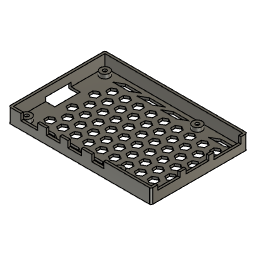
Raspberry pi 4B Case 01 (Autodesk Fusion 360 design; units mm, degrees)
Autodesk Fusion 360 part; units mm, degrees
sketch "スケッチ1" plane through (0, 0, 0) normal (0, 0, 1) x (1, 0, 0)
  line L0 (2.2, 2.2) -> (87.2, 2.2) construction
  line L1 (87.2, 2.2) -> (87.2, 58.2) construction
  line L2 (87.2, 58.2) -> (2.2, 58.2) construction
  line L3 (5.7, 5.7) -> (63.7, 5.7) construction
  line L4 (63.7, 5.7) -> (63.7, 54.7) construction
  line L5 (63.7, 54.7) -> (5.7, 54.7) construction
  line L6 (5.7, 54.7) -> (5.7, 5.7) construction
  circle A0 centre (5.7, 54.7) radius 1.15
  circle A1 centre (63.7, 54.7) radius 1.15
  circle A2 centre (63.7, 5.7) radius 1.15
  circle A3 centre (5.7, 5.7) radius 1.15
  line L7 (2.2, 58.2) -> (2.2, 2.2) construction
  line L8 (0, 0) -> (89.4, 0)
  line L9 (89.4, 0) -> (89.4, 60.4)
  line L10 (89.4, 60.4) -> (0, 60.4)
  line L11 (0, 60.4) -> (0, 0)
  line L12 (1.5, 58.9) -> (87.9, 58.9)
  line L13 (87.9, 58.9) -> (87.9, 1.5)
  line L14 (87.9, 1.5) -> (1.5, 1.5)
  line L15 (1.5, 1.5) -> (1.5, 58.9)
  circle A4 centre (5.7, 54.7) radius 3
  circle A5 centre (63.7, 54.7) radius 3
  circle A6 centre (63.7, 5.7) radius 3
  circle A7 centre (5.7, 5.7) radius 3
  line L16 (8.2, 0.7) -> (17.7, 0.7) construction
  line L17 (17.7, 0.7) -> (17.7, 9.7) construction
  line L18 (17.7, 9.7) -> (8.2, 9.7) construction
  line L19 (8.2, 9.7) -> (8.2, 0.7) construction
  line L20 (7.7, 1.5) -> (7.7, 0)
  line L21 (18.2, 1.5) -> (18.2, 0)
  line L22 (24.2, 0.7) -> (31.7, 0.7) construction
  line L23 (31.7, 0.7) -> (31.7, 9.7) construction
  line L24 (31.7, 9.7) -> (24.2, 9.7) construction
  line L25 (24.2, 9.7) -> (24.2, 0.7) construction
  line L26 (45.2, 0.7) -> (45.2, 9.7) construction
  line L27 (37.7, 0.7) -> (45.2, 0.7) construction
  line L28 (45.2, 9.7) -> (37.7, 9.7) construction
  line L29 (37.7, 9.7) -> (37.7, 0.7) construction
  line L30 (23.7, 1.5) -> (23.7, 0)
  line L31 (37.2, 1.5) -> (37.2, 0)
  line L32 (32.2, 1.5) -> (32.2, 0)
  line L33 (45.7, 1.5) -> (45.7, 0)
  line L34 (52.7, 0.2) -> (59.2, 0.2) construction
  line L35 (59.2, 0.2) -> (59.2, 15.2) construction
  line L36 (59.2, 15.2) -> (52.7, 15.2) construction
  line L37 (52.7, 15.2) -> (52.7, 0.2) construction
  line L38 (90.2, 4.7) -> (72.7, 4.7) construction
  line L39 (90.2, 17.7) -> (90.2, 4.7) construction
  line L40 (72.7, 4.7) -> (72.7, 17.7) construction
  line L41 (72.7, 17.7) -> (90.2, 17.7) construction
  line L42 (90.2, 35.7) -> (72.7, 35.7) construction
  line L43 (90.2, 22.7) -> (90.2, 35.7) construction
  line L44 (72.7, 35.7) -> (72.7, 22.7) construction
  line L45 (72.7, 22.7) -> (90.2, 22.7) construction
  line L46 (52.2, 1.5) -> (52.2, 0)
  line L47 (59.7, 1.5) -> (59.7, 0)
  line L48 (69.2, 39.95) -> (90.2, 39.95) construction
  line L49 (90.2, 55.95) -> (69.2, 55.95) construction
  line L50 (69.2, 55.95) -> (69.2, 39.95) construction
  line L51 (90.2, 39.95) -> (90.2, 55.95) construction
  line L52 (81.45, 17.7) -> (81.45, 4.7) construction
  line L53 (72.7, 11.2) -> (90.2, 11.2) construction
  line L54 (81.45, 35.7) -> (81.45, 22.7) construction
  line L55 (72.7, 29.2) -> (90.2, 29.2) construction
  line L56 (79.7, 55.95) -> (79.7, 39.95) construction
  line L57 (69.2, 47.95) -> (90.2, 47.95) construction
  line L58 (87.9, 4.2) -> (89.4, 4.2)
  line L59 (87.9, 18.2) -> (89.4, 18.2)
  line L60 (87.9, 21.9659) -> (89.4, 21.9659)
  line L61 (87.9, 36.2) -> (89.4, 36.2)
  line L62 (89.4, 39.45) -> (87.9, 39.45)
  line L63 (87.9, 56.45) -> (89.4, 56.45)
  line L64 (4.2, 35.7) -> (15.7, 35.7) construction
  line L65 (15.7, 35.7) -> (15.7, 23.7) construction
  line L66 (15.7, 23.7) -> (4.2, 23.7) construction
  line L67 (4.2, 23.7) -> (4.2, 35.7) construction
  line L68 (0, 37.7) -> (7.2, 37.7)
  line L69 (7.2, 37.7) -> (7.2, 21.7)
  line L70 (7.2, 21.7) -> (0, 21.7)
  circle A8 centre (5.7, 5.7) radius 2
  circle A9 centre (63.7, 5.7) radius 2
  circle A10 centre (63.7, 54.7) radius 2
  circle A11 centre (5.7, 54.7) radius 2
  dimension "d1" = 49
  dimension "d2" = 58
  dimension "d3" = 2.3
  dimension "d5" = 3.5
  dimension "d7" = 56
  dimension "d8" = 85
  dimension "d9" = 3.5
  dimension "d10" = 0.7
  dimension "d11" = 0.7
  dimension "d12" = 0.7
  dimension "d13" = 0.7
  dimension "d14" = 1.5
  dimension "d15" = 1.5
  dimension "d16" = 1.5
  dimension "d17" = 1.5
  dimension "d18" = 6
  dimension "d19" = 6
  dimension "d20" = 15.5
  dimension "d21" = 9
  dimension "d22" = 1.5
  dimension "d23" = 0.5
  dimension "d24" = 0.5
  dimension "d25" = 22
  dimension "d26" = 29.5
  dimension "d27" = 35.5
  dimension "d28" = 43
  dimension "d29" = 1.5
  dimension "d30" = 1.5
  dimension "d31" = 0.5
  dimension "d32" = 0.5
  dimension "d33" = 0.5
  dimension "d34" = 0.5
  dimension "d35" = 50.5
  dimension "d36" = 57
  dimension "d37" = 15
  dimension "d38" = 2
  dimension "d39" = 0.5
  dimension "d40" = 0.5
  dimension "d41" = 6.5
  dimension "d42" = 7.5
  dimension "d43" = 9.5
  dimension "d44" = 7.5
  dimension "d46" = 13
  dimension "d47" = 16
  dimension "d48" = 9
  dimension "d49" = 27
  dimension "d50" = 45.75
  dimension "d51" = 21
  dimension "d52" = 17.5
  dimension "d53" = 3
  dimension "d54" = 3
  dimension "d55" = 3
  dimension "d56" = 0.5
  dimension "d57" = 0.5
  dimension "d58" = 0.5
  dimension "d59" = 0.5
  dimension "d60" = 0.5
  dimension "d61" = 0.7341
  dimension "d62" = 21.5
  dimension "d63" = 11.5
  dimension "d64" = 12
  dimension "d65" = 2
  dimension "d66" = 2
  dimension "d67" = 2
  dimension "d68" = 3
  dimension "d84" = 60.4
  dimension "d85" = 89.4
  dimension "d127" = 4
  constraint horizontal L0
  constraint vertical L1
  constraint horizontal L2
  constraint horizontal L3
  constraint vertical L4
  constraint horizontal L5
  constraint vertical L6
  constraint coincident L5.end L6.start
  constraint coincident L4.end L5.start
  constraint coincident L3.end L4.start
  constraint coincident L3.start L6.end
  constraint equal A0 A3
  constraint equal A0 A1
  constraint equal A1 A2
  constraint vertical L7
  constraint horizontal L8
  constraint vertical L9
  constraint horizontal L10
  constraint vertical L11
  constraint coincident L8.start L11.end
  constraint horizontal L12
  constraint vertical L13
  constraint horizontal L14
  constraint vertical L15
  constraint concentric A0 A4
  constraint concentric A1 A5
  constraint concentric A2 A6
  constraint concentric A3 A7
  constraint equal A4 A7
  constraint equal A4 A5
  constraint equal A5 A6
  constraint horizontal L16
  constraint vertical L17
  constraint horizontal L18
  constraint vertical L19
  constraint coincident L14 L20.start
  constraint coincident L8 L20.end
  constraint perpendicular L8 L20
  constraint coincident L14 L21.start
  constraint coincident L8 L21.end
  constraint perpendicular L8 L21
  constraint horizontal L22
  constraint vertical L23
  constraint horizontal L24
  constraint vertical L25
  constraint horizontal L27
  constraint vertical L26
  constraint horizontal L28
  constraint vertical L29
  constraint equal L17 L23
  constraint equal L23 L26
  constraint coincident L14 L30.start
  constraint coincident L8 L30.end
  constraint perpendicular L8 L30
  constraint coincident L14 L31.start
  constraint coincident L8 L31.end
  constraint perpendicular L8 L31
  constraint coincident L14 L32.start
  constraint coincident L8 L32.end
  constraint perpendicular L14 L32
  constraint coincident L14 L33.start
  constraint coincident L8 L33.end
  constraint perpendicular L8 L33
  constraint horizontal L34
  constraint vertical L35
  constraint horizontal L36
  constraint vertical L37
  constraint horizontal L38
  constraint vertical L40
  constraint horizontal L41
  constraint vertical L39
  constraint horizontal L42
  constraint vertical L44
  constraint horizontal L45
  constraint vertical L43
  constraint coincident L14 L46.start
  constraint coincident L8 L46.end
  constraint perpendicular L8 L46
  constraint coincident L14 L47.start
  constraint coincident L8 L47.end
  constraint perpendicular L8 L47
  constraint horizontal L49
  constraint vertical L50
  constraint horizontal L48
  constraint vertical L51
  constraint midpoint L41 L52.start
  constraint midpoint L38 L52.end
  constraint coincident L40 L53.start
  constraint perpendicular L40 L53
  constraint midpoint L52 L53
  constraint midpoint L42 L54.start
  constraint midpoint L45 L54.end
  constraint coincident L44 L55.start
  constraint coincident L43 L55.end
  constraint perpendicular L43 L55
  constraint midpoint L49 L56.start
  constraint midpoint L48 L56.end
  constraint coincident L50 L57.start
  constraint coincident L51 L57.end
  constraint perpendicular L51 L57
  constraint midpoint L56 L57
  constraint midpoint L54 L55
  constraint equal L40 L44
  constraint equal L41 L45
  constraint coincident L13 L58.start
  constraint coincident L9 L58.end
  constraint perpendicular L9 L58
  constraint coincident L13 L59.start
  constraint coincident L9 L59.end
  constraint perpendicular L9 L59
  constraint coincident L13 L60.start
  constraint coincident L9 L60.end
  constraint perpendicular L9 L60
  constraint coincident L13 L61.start
  constraint coincident L9 L61.end
  constraint perpendicular L9 L61
  constraint coincident L9 L62.start
  constraint coincident L13 L62.end
  constraint perpendicular L9 L62
  constraint coincident L13 L63.start
  constraint coincident L9 L63.end
  constraint perpendicular L9 L63
  constraint horizontal L64
  constraint vertical L65
  constraint horizontal L66
  constraint vertical L67
  constraint coincident L11 L68.start
  constraint perpendicular L15 L68
  constraint perpendicular L66 L69
  constraint coincident L11 L70.end
  constraint perpendicular L11 L70
  constraint concentric A7 A8
  constraint concentric A2 A9
  constraint concentric A5 A10
  constraint concentric A0 A11
  constraint equal A8 A9
  constraint equal A9 A10
  constraint equal A10 A11
  measures "d1" distance of L3.start L5.end
  measures "d2" distance of L4.end L5.end
  measures "d3" diameter of A0
  measures "d5" distance of L2 L5
  measures "d7" distance of L0.end L1.end
  measures "d8" distance of L0.end L0.start
  measures "d9" distance of L6 L7
  measures "d10" distance of L2 L12
  measures "d11" distance of L7 L15
  measures "d12" distance of L0 L14
  measures "d13" distance of L1 L13
  measures "d14" distance of L10 L12
  measures "d15" distance of L11 L15
  measures "d16" distance of L9 L13
  measures "d17" distance of L8 L14
  measures "d18" diameter of A4
  measures "d19" distance of L7 L19
  measures "d20" distance of L7 L17
  measures "d21" distance of L16.end L17.end
  measures "d22" distance of L0 L16
  measures "d23" distance of L19 L20
  measures "d24" distance of L17 L21
  measures "d25" distance of L7 L25
  measures "d26" distance of L7 L23
  measures "d27" distance of L7 L29
  measures "d28" distance of L7 L26
  measures "d29" distance of L0 L22
  measures "d30" distance of L0 L27
  measures "d31" distance of L25 L30.start
  measures "d32" distance of L23 L32.start
  measures "d33" distance of L29 L31.start
  measures "d34" distance of L26 L33.start
  measures "d35" distance of L7 L37
  measures "d36" distance of L7 L35
  measures "d37" distance of L34.end L35.end
  measures "d38" distance of L0 L34
  measures "d39" distance of L37 L46
  measures "d40" distance of L35 L47
  measures "d41" distance of L35 L37
  measures "d42" distance of L26 L29
  measures "d43" distance of L17 L19
  measures "d44" distance of L23 L25
  measures "d46" distance of L42 L45
  measures "d47" distance of L48 L49
  measures "d48" distance of L0 L53
  measures "d49" distance of L0 L55
  measures "d50" distance of L0 L57
  measures "d51" distance of L49.start L49.end
  measures "d52" distance of L42.end L42.start
  measures "d53" distance of L1 L39
  measures "d54" distance of L1 L43
  measures "d55" distance of L1 L51
  measures "d56" distance of L41 L59
  measures "d57" distance of L38 L58
  measures "d58" distance of L49 L63
  measures "d59" distance of L48 L62
  measures "d60" distance of L42 L61
  measures "d61" distance of L45 L60
  measures "d62" distance of L0 L66
  measures "d63" distance of L65.end L66.end
  measures "d64" distance of L64 L66
  measures "d65" distance of L7 L67
  measures "d66" distance of L64 L68
  measures "d67" distance of L66 L70
  measures "d68" distance of L67 L69
  measures "d84" distance of L8 L10
  measures "d85" distance of L9 L11
  measures "d127" diameter of A11
extrude "押し出し1" add sketch "スケッチ1" along normal blind 1.5 contours L8 L11 L14 L15 L20 L70 | L8 L14 L20 L21 | L8 L14 L21 L30 | L12 L13 L14 L15 L68 L69 L70 | L9 L10 L11 L12 L13 L15 L63 L68 | L8 L14 L30 L32 | L8 L14 L31 L32 | L8 L14 L31 L33 | L9 L13 L62 L63 | L8 L14 L33 L46 | L9 L13 L61 L62 | L8 L14 L46 L47 | L9 L13 L60 L61 | L8 L9 L13 L14 L47 L58 | L9 L13 L59 L60 | L9 L13 L58 L59 | A4 | A5 | A6 | A7 | A8 | A9 | A10 | A11
extrude "押し出し2" add sketch "スケッチ1" along normal blind 4 contours A4 | A5 | A6 | A7 | A8 | A9 | A10 | A11
extrude "押し出し3" add sketch "スケッチ1" along normal blind 5 contours L8 L11 L14 L15 L20 L70 | L8 L14 L20 L21 | L8 L14 L21 L30 | L9 L10 L11 L12 L13 L15 L63 L68 | L8 L14 L30 L32 | L8 L14 L31 L32 | L8 L14 L31 L33 | L9 L13 L62 L63 | L8 L14 L33 L46 | L9 L13 L61 L62 | L8 L14 L46 L47 | L9 L13 L60 L61 | L8 L9 L13 L14 L47 L58 | L9 L13 L59 L60 | L9 L13 L58 L59
extrude "押し出し4" add sketch "スケッチ1" along normal blind 6 contours L8 L11 L14 L15 L20 L70 | L8 L14 L21 L30 | L9 L10 L11 L12 L13 L15 L63 L68 | L8 L14 L31 L32 | L8 L14 L33 L46 | L9 L13 L61 L62 | L9 L13 L60 L61 | L8 L9 L13 L14 L47 L58 | L9 L13 L59 L60 | L9 L13 L58 L59
extrude "押し出し5" add sketch "スケッチ1" along normal blind 5 from surface at 4 contours L11 L15 L68 L70
extrude "押し出し6" add sketch "スケッチ1" along normal blind 9 contours L8 L11 L14 L15 L20 L70 | L8 L14 L21 L30 | L9 L10 L11 L12 L13 L15 L63 L68 | L8 L14 L31 L32 | L8 L14 L33 L46 | L9 L13 L61 L62 | L8 L9 L13 L14 L47 L58 | L9 L13 L59 L60
fillet "フィレット1" radius 1 4 edges at (89.4, 60.4, 4.5) (89.4, 0, 4.5) (0, 60.4, 4.5) (0, 0, 4.5)
sketch "スケッチ2" plane through (0, 0, 0) normal (0, 0, 1) x (1, 0, 0)
  line L0 (0, 0) -> (89.4, 0) construction
  line L1 (89.4, 0) -> (89.4, 60.4) construction
  line L2 (89.4, 60.4) -> (0, 60.4) construction
  line L3 (0, 60.4) -> (0, 0) construction
  line L4 (10.5, 11.5566) -> (13, 10.1132)
  line L5 (10.5, 14.4434) -> (10.5, 11.5566)
  line L6 (15.5, 11.5566) -> (15.5, 14.4434)
  line L7 (13, 10.1132) -> (15.5, 11.5566)
  line L8 (15.5, 14.4434) -> (13, 15.8868)
  line L9 (13, 15.8868) -> (10.5, 14.4434)
  line L10 (17, 22.8868) -> (14.5, 21.4434)
  line L11 (14.5, 18.5566) -> (17, 17.1132)
  line L12 (14.5, 18.5566) -> (17, 17.1132)
  line L13 (19.5, 18.5566) -> (19.5, 21.4434)
  line L14 (14.5, 21.4434) -> (14.5, 18.5566)
  line L15 (19.5, 21.4434) -> (17, 22.8868)
  line L16 (17, 22.8868) -> (14.5, 21.4434)
  line L17 (14.5, 21.4434) -> (14.5, 18.5566)
  line L18 (17, 17.1132) -> (19.5, 18.5566)
  line L19 (19.5, 18.5566) -> (19.5, 21.4434)
  line L20 (19.5, 21.4434) -> (17, 22.8868)
  line L21 (17, 17.1132) -> (19.5, 18.5566)
  line L22 (13, 13) -> (17, 13) construction
  line L23 (17, 13) -> (17, 20) construction
  line L24 (17, 20) -> (13, 20) construction
  line L25 (13, 20) -> (13, 13) construction
  line L26 (21.125, 10.1132) -> (23.625, 11.5566)
  line L27 (18.625, 11.5566) -> (21.125, 10.1132)
  line L28 (18.625, 14.4434) -> (18.625, 11.5566)
  line L29 (21.125, 15.8868) -> (18.625, 14.4434)
  line L30 (23.625, 14.4434) -> (21.125, 15.8868)
  line L31 (23.625, 11.5566) -> (23.625, 14.4434)
  line L32 (22.625, 18.5566) -> (25.125, 17.1132)
  line L33 (22.625, 21.4434) -> (22.625, 18.5566)
  line L34 (25.125, 22.8868) -> (22.625, 21.4434)
  line L35 (27.625, 21.4434) -> (25.125, 22.8868)
  line L36 (27.625, 18.5566) -> (27.625, 21.4434)
  line L37 (25.125, 17.1132) -> (27.625, 18.5566)
  line L38 (29.25, 10.1132) -> (31.75, 11.5566)
  line L39 (26.75, 11.5566) -> (29.25, 10.1132)
  line L40 (26.75, 14.4434) -> (26.75, 11.5566)
  line L41 (29.25, 15.8868) -> (26.75, 14.4434)
  line L42 (31.75, 14.4434) -> (29.25, 15.8868)
  line L43 (31.75, 11.5566) -> (31.75, 14.4434)
  line L44 (30.75, 18.5566) -> (33.25, 17.1132)
  line L45 (30.75, 21.4434) -> (30.75, 18.5566)
  line L46 (33.25, 22.8868) -> (30.75, 21.4434)
  line L47 (35.75, 21.4434) -> (33.25, 22.8868)
  line L48 (35.75, 18.5566) -> (35.75, 21.4434)
  line L49 (33.25, 17.1132) -> (35.75, 18.5566)
  line L50 (37.375, 10.1132) -> (39.875, 11.5566)
  line L51 (34.875, 11.5566) -> (37.375, 10.1132)
  line L52 (34.875, 14.4434) -> (34.875, 11.5566)
  line L53 (37.375, 15.8868) -> (34.875, 14.4434)
  line L54 (39.875, 14.4434) -> (37.375, 15.8868)
  line L55 (39.875, 11.5566) -> (39.875, 14.4434)
  line L56 (38.875, 18.5566) -> (41.375, 17.1132)
  line L57 (38.875, 21.4434) -> (38.875, 18.5566)
  line L58 (41.375, 22.8868) -> (38.875, 21.4434)
  line L59 (43.875, 21.4434) -> (41.375, 22.8868)
  line L60 (43.875, 18.5566) -> (43.875, 21.4434)
  line L61 (41.375, 17.1132) -> (43.875, 18.5566)
  line L62 (45.5, 10.1132) -> (48, 11.5566)
  line L63 (43, 11.5566) -> (45.5, 10.1132)
  line L64 (43, 14.4434) -> (43, 11.5566)
  line L65 (45.5, 15.8868) -> (43, 14.4434)
  line L66 (48, 14.4434) -> (45.5, 15.8868)
  line L67 (48, 11.5566) -> (48, 14.4434)
  line L68 (47, 18.5566) -> (49.5, 17.1132)
  line L69 (47, 21.4434) -> (47, 18.5566)
  line L70 (49.5, 22.8868) -> (47, 21.4434)
  line L71 (52, 21.4434) -> (49.5, 22.8868)
  line L72 (52, 18.5566) -> (52, 21.4434)
  line L73 (49.5, 17.1132) -> (52, 18.5566)
  line L74 (53.625, 10.1132) -> (56.125, 11.5566)
  line L75 (51.125, 11.5566) -> (53.625, 10.1132)
  line L76 (51.125, 14.4434) -> (51.125, 11.5566)
  line L77 (53.625, 15.8868) -> (51.125, 14.4434)
  line L78 (56.125, 14.4434) -> (53.625, 15.8868)
  line L79 (56.125, 11.5566) -> (56.125, 14.4434)
  line L80 (55.125, 18.5566) -> (57.625, 17.1132)
  line L81 (55.125, 21.4434) -> (55.125, 18.5566)
  line L82 (57.625, 22.8868) -> (55.125, 21.4434)
  line L83 (60.125, 21.4434) -> (57.625, 22.8868)
  line L84 (60.125, 18.5566) -> (60.125, 21.4434)
  line L85 (57.625, 17.1132) -> (60.125, 18.5566)
  line L86 (61.75, 10.1132) -> (64.25, 11.5566)
  line L87 (59.25, 11.5566) -> (61.75, 10.1132)
  line L88 (59.25, 14.4434) -> (59.25, 11.5566)
  line L89 (61.75, 15.8868) -> (59.25, 14.4434)
  line L90 (64.25, 14.4434) -> (61.75, 15.8868)
  line L91 (64.25, 11.5566) -> (64.25, 14.4434)
  line L92 (63.25, 18.5566) -> (65.75, 17.1132)
  line L93 (63.25, 21.4434) -> (63.25, 18.5566)
  line L94 (65.75, 22.8868) -> (63.25, 21.4434)
  line L95 (68.25, 21.4434) -> (65.75, 22.8868)
  line L96 (68.25, 18.5566) -> (68.25, 21.4434)
  line L97 (65.75, 17.1132) -> (68.25, 18.5566)
  line L98 (69.875, 10.1132) -> (72.375, 11.5566)
  line L99 (67.375, 11.5566) -> (69.875, 10.1132)
  line L100 (67.375, 14.4434) -> (67.375, 11.5566)
  line L101 (69.875, 15.8868) -> (67.375, 14.4434)
  line L102 (72.375, 14.4434) -> (69.875, 15.8868)
  line L103 (72.375, 11.5566) -> (72.375, 14.4434)
  line L104 (71.375, 18.5566) -> (73.875, 17.1132)
  line L105 (71.375, 21.4434) -> (71.375, 18.5566)
  line L106 (73.875, 22.8868) -> (71.375, 21.4434)
  line L107 (76.375, 21.4434) -> (73.875, 22.8868)
  line L108 (76.375, 18.5566) -> (76.375, 21.4434)
  line L109 (73.875, 17.1132) -> (76.375, 18.5566)
  line L110 (78, 10.1132) -> (80.5, 11.5566)
  line L111 (75.5, 11.5566) -> (78, 10.1132)
  line L112 (75.5, 14.4434) -> (75.5, 11.5566)
  line L113 (78, 15.8868) -> (75.5, 14.4434)
  line L114 (80.5, 14.4434) -> (78, 15.8868)
  line L115 (80.5, 11.5566) -> (80.5, 14.4434)
  line L116 (79.5, 18.5566) -> (82, 17.1132)
  line L117 (79.5, 21.4434) -> (79.5, 18.5566)
  line L118 (82, 22.8868) -> (79.5, 21.4434)
  line L119 (84.5, 21.4434) -> (82, 22.8868)
  line L120 (84.5, 18.5566) -> (84.5, 21.4434)
  line L121 (82, 17.1132) -> (84.5, 18.5566)
  line L122 (13, 24.1132) -> (15.5, 25.5566)
  line L123 (10.5, 25.5566) -> (13, 24.1132)
  line L124 (10.5, 28.4434) -> (10.5, 25.5566)
  line L125 (13, 29.8868) -> (10.5, 28.4434)
  line L126 (15.5, 28.4434) -> (13, 29.8868)
  line L127 (15.5, 25.5566) -> (15.5, 28.4434)
  line L128 (14.5, 32.5566) -> (17, 31.1132)
  line L129 (14.5, 35.4434) -> (14.5, 32.5566)
  line L130 (17, 36.8868) -> (14.5, 35.4434)
  line L131 (19.5, 35.4434) -> (17, 36.8868)
  line L132 (19.5, 32.5566) -> (19.5, 35.4434)
  line L133 (17, 31.1132) -> (19.5, 32.5566)
  line L134 (21.125, 24.1132) -> (23.625, 25.5566)
  line L135 (18.625, 25.5566) -> (21.125, 24.1132)
  line L136 (18.625, 28.4434) -> (18.625, 25.5566)
  line L137 (21.125, 29.8868) -> (18.625, 28.4434)
  line L138 (23.625, 28.4434) -> (21.125, 29.8868)
  line L139 (23.625, 25.5566) -> (23.625, 28.4434)
  line L140 (22.625, 32.5566) -> (25.125, 31.1132)
  line L141 (22.625, 35.4434) -> (22.625, 32.5566)
  line L142 (25.125, 36.8868) -> (22.625, 35.4434)
  line L143 (27.625, 35.4434) -> (25.125, 36.8868)
  line L144 (27.625, 32.5566) -> (27.625, 35.4434)
  line L145 (25.125, 31.1132) -> (27.625, 32.5566)
  line L146 (29.25, 24.1132) -> (31.75, 25.5566)
  line L147 (26.75, 25.5566) -> (29.25, 24.1132)
  line L148 (26.75, 28.4434) -> (26.75, 25.5566)
  line L149 (29.25, 29.8868) -> (26.75, 28.4434)
  line L150 (31.75, 28.4434) -> (29.25, 29.8868)
  line L151 (31.75, 25.5566) -> (31.75, 28.4434)
  line L152 (30.75, 32.5566) -> (33.25, 31.1132)
  line L153 (30.75, 35.4434) -> (30.75, 32.5566)
  line L154 (33.25, 36.8868) -> (30.75, 35.4434)
  line L155 (35.75, 35.4434) -> (33.25, 36.8868)
  line L156 (35.75, 32.5566) -> (35.75, 35.4434)
  line L157 (33.25, 31.1132) -> (35.75, 32.5566)
  line L158 (37.375, 24.1132) -> (39.875, 25.5566)
  line L159 (34.875, 25.5566) -> (37.375, 24.1132)
  line L160 (34.875, 28.4434) -> (34.875, 25.5566)
  line L161 (37.375, 29.8868) -> (34.875, 28.4434)
  line L162 (39.875, 28.4434) -> (37.375, 29.8868)
  line L163 (39.875, 25.5566) -> (39.875, 28.4434)
  line L164 (38.875, 32.5566) -> (41.375, 31.1132)
  line L165 (38.875, 35.4434) -> (38.875, 32.5566)
  line L166 (41.375, 36.8868) -> (38.875, 35.4434)
  line L167 (43.875, 35.4434) -> (41.375, 36.8868)
  line L168 (43.875, 32.5566) -> (43.875, 35.4434)
  line L169 (41.375, 31.1132) -> (43.875, 32.5566)
  line L170 (45.5, 24.1132) -> (48, 25.5566)
  line L171 (43, 25.5566) -> (45.5, 24.1132)
  line L172 (43, 28.4434) -> (43, 25.5566)
  line L173 (45.5, 29.8868) -> (43, 28.4434)
  line L174 (48, 28.4434) -> (45.5, 29.8868)
  line L175 (48, 25.5566) -> (48, 28.4434)
  line L176 (47, 32.5566) -> (49.5, 31.1132)
  line L177 (47, 35.4434) -> (47, 32.5566)
  line L178 (49.5, 36.8868) -> (47, 35.4434)
  line L179 (52, 35.4434) -> (49.5, 36.8868)
  line L180 (52, 32.5566) -> (52, 35.4434)
  line L181 (49.5, 31.1132) -> (52, 32.5566)
  line L182 (53.625, 24.1132) -> (56.125, 25.5566)
  line L183 (51.125, 25.5566) -> (53.625, 24.1132)
  line L184 (51.125, 28.4434) -> (51.125, 25.5566)
  line L185 (53.625, 29.8868) -> (51.125, 28.4434)
  line L186 (56.125, 28.4434) -> (53.625, 29.8868)
  line L187 (56.125, 25.5566) -> (56.125, 28.4434)
  line L188 (55.125, 32.5566) -> (57.625, 31.1132)
  line L189 (55.125, 35.4434) -> (55.125, 32.5566)
  line L190 (57.625, 36.8868) -> (55.125, 35.4434)
  line L191 (60.125, 35.4434) -> (57.625, 36.8868)
  line L192 (60.125, 32.5566) -> (60.125, 35.4434)
  line L193 (57.625, 31.1132) -> (60.125, 32.5566)
  line L194 (61.75, 24.1132) -> (64.25, 25.5566)
  line L195 (59.25, 25.5566) -> (61.75, 24.1132)
  line L196 (59.25, 28.4434) -> (59.25, 25.5566)
  line L197 (61.75, 29.8868) -> (59.25, 28.4434)
  line L198 (64.25, 28.4434) -> (61.75, 29.8868)
  line L199 (64.25, 25.5566) -> (64.25, 28.4434)
  line L200 (63.25, 32.5566) -> (65.75, 31.1132)
  line L201 (63.25, 35.4434) -> (63.25, 32.5566)
  line L202 (65.75, 36.8868) -> (63.25, 35.4434)
  line L203 (68.25, 35.4434) -> (65.75, 36.8868)
  line L204 (68.25, 32.5566) -> (68.25, 35.4434)
  line L205 (65.75, 31.1132) -> (68.25, 32.5566)
  line L206 (69.875, 24.1132) -> (72.375, 25.5566)
  line L207 (67.375, 25.5566) -> (69.875, 24.1132)
  line L208 (67.375, 28.4434) -> (67.375, 25.5566)
  line L209 (69.875, 29.8868) -> (67.375, 28.4434)
  line L210 (72.375, 28.4434) -> (69.875, 29.8868)
  line L211 (72.375, 25.5566) -> (72.375, 28.4434)
  line L212 (71.375, 32.5566) -> (73.875, 31.1132)
  line L213 (71.375, 35.4434) -> (71.375, 32.5566)
  line L214 (73.875, 36.8868) -> (71.375, 35.4434)
  line L215 (76.375, 35.4434) -> (73.875, 36.8868)
  line L216 (76.375, 32.5566) -> (76.375, 35.4434)
  line L217 (73.875, 31.1132) -> (76.375, 32.5566)
  line L218 (78, 24.1132) -> (80.5, 25.5566)
  line L219 (75.5, 25.5566) -> (78, 24.1132)
  line L220 (75.5, 28.4434) -> (75.5, 25.5566)
  line L221 (78, 29.8868) -> (75.5, 28.4434)
  line L222 (80.5, 28.4434) -> (78, 29.8868)
  line L223 (80.5, 25.5566) -> (80.5, 28.4434)
  line L224 (79.5, 32.5566) -> (82, 31.1132)
  line L225 (79.5, 35.4434) -> (79.5, 32.5566)
  line L226 (82, 36.8868) -> (79.5, 35.4434)
  line L227 (84.5, 35.4434) -> (82, 36.8868)
  line L228 (84.5, 32.5566) -> (84.5, 35.4434)
  line L229 (82, 31.1132) -> (84.5, 32.5566)
  line L230 (13, 38.1132) -> (15.5, 39.5566)
  line L231 (10.5, 39.5566) -> (13, 38.1132)
  line L232 (10.5, 42.4434) -> (10.5, 39.5566)
  line L233 (13, 43.8868) -> (10.5, 42.4434)
  line L234 (15.5, 42.4434) -> (13, 43.8868)
  line L235 (15.5, 39.5566) -> (15.5, 42.4434)
  line L236 (14.5, 46.5566) -> (17, 45.1132)
  line L237 (14.5, 49.4434) -> (14.5, 46.5566)
  line L238 (17, 50.8868) -> (14.5, 49.4434)
  line L239 (19.5, 49.4434) -> (17, 50.8868)
  line L240 (19.5, 46.5566) -> (19.5, 49.4434)
  line L241 (17, 45.1132) -> (19.5, 46.5566)
  line L242 (21.125, 38.1132) -> (23.625, 39.5566)
  line L243 (18.625, 39.5566) -> (21.125, 38.1132)
  line L244 (18.625, 42.4434) -> (18.625, 39.5566)
  line L245 (21.125, 43.8868) -> (18.625, 42.4434)
  line L246 (23.625, 42.4434) -> (21.125, 43.8868)
  line L247 (23.625, 39.5566) -> (23.625, 42.4434)
  line L248 (22.625, 46.5566) -> (25.125, 45.1132)
  line L249 (22.625, 49.4434) -> (22.625, 46.5566)
  line L250 (25.125, 50.8868) -> (22.625, 49.4434)
  line L251 (27.625, 49.4434) -> (25.125, 50.8868)
  line L252 (27.625, 46.5566) -> (27.625, 49.4434)
  line L253 (25.125, 45.1132) -> (27.625, 46.5566)
  line L254 (29.25, 38.1132) -> (31.75, 39.5566)
  line L255 (26.75, 39.5566) -> (29.25, 38.1132)
  line L256 (26.75, 42.4434) -> (26.75, 39.5566)
  line L257 (29.25, 43.8868) -> (26.75, 42.4434)
  line L258 (31.75, 42.4434) -> (29.25, 43.8868)
  line L259 (31.75, 39.5566) -> (31.75, 42.4434)
  line L260 (30.75, 46.5566) -> (33.25, 45.1132)
  line L261 (30.75, 49.4434) -> (30.75, 46.5566)
  line L262 (33.25, 50.8868) -> (30.75, 49.4434)
  line L263 (35.75, 49.4434) -> (33.25, 50.8868)
  line L264 (35.75, 46.5566) -> (35.75, 49.4434)
  line L265 (33.25, 45.1132) -> (35.75, 46.5566)
  line L266 (37.375, 38.1132) -> (39.875, 39.5566)
  line L267 (34.875, 39.5566) -> (37.375, 38.1132)
  line L268 (34.875, 42.4434) -> (34.875, 39.5566)
  line L269 (37.375, 43.8868) -> (34.875, 42.4434)
  line L270 (39.875, 42.4434) -> (37.375, 43.8868)
  line L271 (39.875, 39.5566) -> (39.875, 42.4434)
  line L272 (38.875, 46.5566) -> (41.375, 45.1132)
  line L273 (38.875, 49.4434) -> (38.875, 46.5566)
  line L274 (41.375, 50.8868) -> (38.875, 49.4434)
  line L275 (43.875, 49.4434) -> (41.375, 50.8868)
  line L276 (43.875, 46.5566) -> (43.875, 49.4434)
  line L277 (41.375, 45.1132) -> (43.875, 46.5566)
  line L278 (45.5, 38.1132) -> (48, 39.5566)
  line L279 (43, 39.5566) -> (45.5, 38.1132)
  line L280 (43, 42.4434) -> (43, 39.5566)
  line L281 (45.5, 43.8868) -> (43, 42.4434)
  line L282 (48, 42.4434) -> (45.5, 43.8868)
  line L283 (48, 39.5566) -> (48, 42.4434)
  line L284 (47, 46.5566) -> (49.5, 45.1132)
  line L285 (47, 49.4434) -> (47, 46.5566)
  line L286 (49.5, 50.8868) -> (47, 49.4434)
  line L287 (52, 49.4434) -> (49.5, 50.8868)
  line L288 (52, 46.5566) -> (52, 49.4434)
  line L289 (49.5, 45.1132) -> (52, 46.5566)
  line L290 (53.625, 38.1132) -> (56.125, 39.5566)
  line L291 (51.125, 39.5566) -> (53.625, 38.1132)
  line L292 (51.125, 42.4434) -> (51.125, 39.5566)
  line L293 (53.625, 43.8868) -> (51.125, 42.4434)
  line L294 (56.125, 42.4434) -> (53.625, 43.8868)
  line L295 (56.125, 39.5566) -> (56.125, 42.4434)
  line L296 (55.125, 46.5566) -> (57.625, 45.1132)
  line L297 (55.125, 49.4434) -> (55.125, 46.5566)
  line L298 (57.625, 50.8868) -> (55.125, 49.4434)
  line L299 (60.125, 49.4434) -> (57.625, 50.8868)
  line L300 (60.125, 46.5566) -> (60.125, 49.4434)
  line L301 (57.625, 45.1132) -> (60.125, 46.5566)
  line L302 (61.75, 38.1132) -> (64.25, 39.5566)
  line L303 (59.25, 39.5566) -> (61.75, 38.1132)
  line L304 (59.25, 42.4434) -> (59.25, 39.5566)
  line L305 (61.75, 43.8868) -> (59.25, 42.4434)
  line L306 (64.25, 42.4434) -> (61.75, 43.8868)
  line L307 (64.25, 39.5566) -> (64.25, 42.4434)
  line L308 (63.25, 46.5566) -> (65.75, 45.1132)
  line L309 (63.25, 49.4434) -> (63.25, 46.5566)
  line L310 (65.75, 50.8868) -> (63.25, 49.4434)
  line L311 (68.25, 49.4434) -> (65.75, 50.8868)
  line L312 (68.25, 46.5566) -> (68.25, 49.4434)
  line L313 (65.75, 45.1132) -> (68.25, 46.5566)
  line L314 (69.875, 38.1132) -> (72.375, 39.5566)
  line L315 (67.375, 39.5566) -> (69.875, 38.1132)
  line L316 (67.375, 42.4434) -> (67.375, 39.5566)
  line L317 (69.875, 43.8868) -> (67.375, 42.4434)
  line L318 (72.375, 42.4434) -> (69.875, 43.8868)
  line L319 (72.375, 39.5566) -> (72.375, 42.4434)
  line L320 (71.375, 46.5566) -> (73.875, 45.1132)
  line L321 (71.375, 49.4434) -> (71.375, 46.5566)
  line L322 (73.875, 50.8868) -> (71.375, 49.4434)
  line L323 (76.375, 49.4434) -> (73.875, 50.8868)
  line L324 (76.375, 46.5566) -> (76.375, 49.4434)
  line L325 (73.875, 45.1132) -> (76.375, 46.5566)
  line L326 (78, 38.1132) -> (80.5, 39.5566)
  line L327 (75.5, 39.5566) -> (78, 38.1132)
  line L328 (75.5, 42.4434) -> (75.5, 39.5566)
  line L329 (78, 43.8868) -> (75.5, 42.4434)
  line L330 (80.5, 42.4434) -> (78, 43.8868)
  line L331 (80.5, 39.5566) -> (80.5, 42.4434)
  line L332 (79.5, 46.5566) -> (82, 45.1132)
  line L333 (79.5, 49.4434) -> (79.5, 46.5566)
  line L334 (82, 50.8868) -> (79.5, 49.4434)
  line L335 (84.5, 49.4434) -> (82, 50.8868)
  line L336 (84.5, 46.5566) -> (84.5, 49.4434)
  line L337 (82, 45.1132) -> (84.5, 46.5566)
  line L338 (0, 6.7929) -> (89.4, 6.7929) construction
  line L339 (0, 54.5395) -> (89.4, 54.5395) construction
  point P0 (13, 13)
  point P1 (17, 20)
  point P2 (17, 20)
  dimension "d86" = 89.4
  dimension "d87" = 60.4
  dimension "d89" = 2.5
  dimension "d90" = 2.5
  dimension "d91" = 2.5
  dimension "d92" = 13
  dimension "d93" = 13
  dimension "d94" = 7
  dimension "d95" = 4
  dimension "d98" = 65
  dimension "d99" = 28
  constraint horizontal L0
  constraint vertical L1
  constraint horizontal L2
  constraint vertical L3
  constraint coincident L0.start L3.end
  constraint vertical L6
  constraint vertical L13
  constraint vertical L19
  constraint coincident P2 P1
  constraint horizontal L22
  constraint vertical L23
  constraint horizontal L24
  constraint vertical L25
  constraint coincident P0 L22.start
  constraint coincident L3 L338.start
  constraint coincident L1 L338.end
  constraint perpendicular L1 L338
  constraint coincident L3 L339.start
  constraint coincident L1 L339.end
  constraint perpendicular L1 L339
  measures "d86" distance of L0.start L0.end
  measures "d87" distance of L0.end L1.end
  measures "d89" distance of P0 L8
  measures "d90" distance of P2 L20
  measures "d91" distance of P2 L15
  measures "d92" distance of L0 P0
  measures "d93" distance of L3 P0
  measures "d94" distance of P0 L24.end
  measures "d95" distance of P2 L24.end
extrude "押し出し7" cut sketch "スケッチ2" along normal up to surface (1.5 mm away)
sketch "スケッチ3" plane through (0, 0, 0) normal (0, 0, 1) x (1, 0, 0)
  line L0 (0, 0) -> (89.4, 0) construction
  line L1 (89.4, 0) -> (89.4, 60.4) construction
  line L2 (89.4, 60.4) -> (0, 60.4) construction
  line L3 (0, 60.4) -> (0, 0) construction
  line L4 (0, 7) -> (89.4, 7) construction
  line L5 (0, 30.2) -> (89.4, 30.2) construction
  line L6 (12, 7) -> (17, 4.1132)
  line L7 (17, 4.1132) -> (27, 4.1132)
  line L8 (27, 4.1132) -> (22, 7)
  line L9 (12, 7) -> (22, 7)
  line L10 (27, 7) -> (37, 7)
  line L11 (27, 7) -> (32, 4.1132)
  line L12 (32, 4.1132) -> (42, 4.1132)
  line L13 (42, 4.1132) -> (37, 7)
  line L14 (42, 7) -> (52, 7)
  line L15 (42, 7) -> (47, 4.1132)
  line L16 (47, 4.1132) -> (57, 4.1132)
  line L17 (57, 4.1132) -> (52, 7)
  line L18 (66.2981, 30.2) -> (66.2981, 0) construction
  line L19 (66.2981, 30.2) -> (66.2981, 60.4) construction
  line L20 (77, 4.1132) -> (87, 4.1132)
  line L21 (72, 7) -> (77, 4.1132)
  line L22 (87, 4.1132) -> (82, 7)
  line L23 (72, 7) -> (82, 7)
  line L24 (27, 53.4) -> (32, 56.2868)
  line L25 (27, 53.4) -> (37, 53.4)
  line L26 (32, 56.2868) -> (42, 56.2868)
  line L27 (72, 53.4) -> (82, 53.4)
  line L28 (27, 56.2868) -> (22, 53.4)
  line L29 (77, 56.2868) -> (87, 56.2868)
  line L30 (87, 56.2868) -> (82, 53.4)
  line L31 (12, 53.4) -> (17, 56.2868)
  line L32 (42, 53.4) -> (52, 53.4)
  line L33 (42, 56.2868) -> (37, 53.4)
  line L34 (17, 56.2868) -> (27, 56.2868)
  line L35 (57, 56.2868) -> (52, 53.4)
  line L36 (12, 53.4) -> (22, 53.4)
  line L37 (72, 53.4) -> (77, 56.2868)
  line L38 (42, 53.4) -> (47, 56.2868)
  line L39 (47, 56.2868) -> (57, 56.2868)
  dimension "d107" = 89.4
  dimension "d108" = 60.4
  dimension "d109" = 12
  dimension "d110" = 30
  dimension "d113" = 150
  dimension "d114" = 10
  dimension "d115" = 5
  dimension "d116" = 7
  dimension "d119" = 30
  dimension "d120" = 0
  dimension "d123" = 30
  dimension "d124" = 0
  constraint horizontal L0
  constraint vertical L1
  constraint vertical L3
  constraint coincident L0.start L3.end
  constraint coincident L3 L4.start
  constraint coincident L1 L4.end
  constraint perpendicular L1 L4
  constraint coincident L3 L5.start
  constraint coincident L1 L5.end
  constraint perpendicular L1 L5
  constraint coincident L4 L6.start
  constraint parallel L4 L7
  constraint coincident L4 L8.end
  constraint coincident L5 L18.start
  constraint coincident L0 L18.end
  constraint perpendicular L0 L18
  constraint coincident L2 L19.end
  constraint perpendicular L2 L19
  constraint equal L18 L19
  constraint symmetric L5 L6.start L31.start
  constraint symmetric L5 L6.end L31.end
  constraint symmetric L5 L7.end L28.start
  constraint symmetric L5 L8.end L28.end
  constraint symmetric L5 L10.start L24.start
  constraint symmetric L5 L10.end L25.end
  constraint symmetric L5 L11.end L24.end
  constraint symmetric L5 L12.end L26.end
  constraint symmetric L5 L14.start L32.start
  constraint symmetric L5 L14.end L32.end
  constraint symmetric L5 L15.end L38.end
  constraint symmetric L5 L16.end L35.start
  constraint symmetric L5 L20.start L29.start
  constraint symmetric L5 L20.end L29.end
  constraint symmetric L5 L21.start L27.start
  constraint symmetric L5 L22.end L27.end
  constraint horizontal L2
  measures "d107" distance of L0.start L0.end
  measures "d108" distance of L0.end L1.end
  measures "d109" distance of L4.start L6.start
  measures "d110" angle of L4 L6
  measures "d113" angle of L4 L8
  measures "d114" distance of L6.end L7.end
  measures "d115" horizontal distance of L6.start L6.end
  measures "d116" distance of L0 L4
extrude "押し出し8" cut sketch "スケッチ3" along normal up to surface (1.5 mm away)
extrude "押し出し9" cut sketch "スケッチ1" along normal blind 2.8 contours A8 | A9 | A10 | A11
chamfer "面取り1" distance 0.7 angle 45 4 edges at (3.8353, 4.9768, 2.8) (61.8353, 4.9768, 2.8) (61.8353, 53.9768, 2.8) (3.8353, 53.9768, 2.8)
